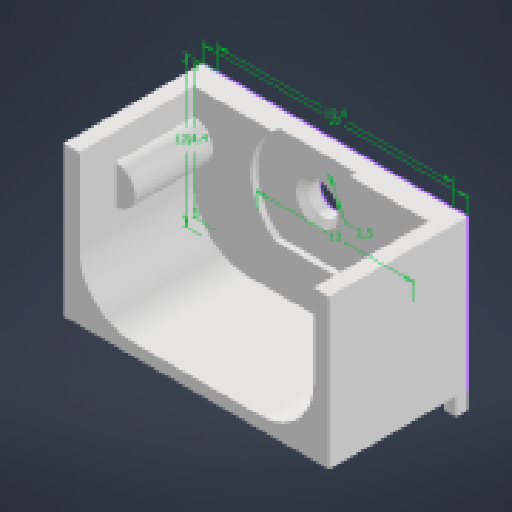
# Autodesk Inventor part: MotorHolder
Saved by Autodesk Inventor 2024 (Build 280153000, 153)
## iProperties
Created: 2023-10-23
Part Number: MotorHolder
Material: Generic
Document SubType Name: Modeling
Designer: 21guslof
Density: 1 g/cm^3
Appearance: Default
Author: 21guslof
Autodesk Inventor part; units mm, degrees
ref_plane "YZ Plane" through (0, 0, 0) normal (1, 0, 0) x (0, 1, 0)
ref_plane "XZ Plane" through (0, 0, 0) normal (0, 1, 0) x (-1, 0, 0)
ref_plane "XY Plane" through (0, 0, 0) normal (0, 0, 1) x (1, 0, 0)
sketch "Sketch1" plane through (0, 0, 0) normal (0, 0, 1) x (1, 0, 0)
  line L0 (9.7, 0) -> (-9.7, 0)
  line L1 (-9.7, 0) -> (-9.7, 11.4)
  line L2 (-9.7, 11.4) -> (9.7, 11.4)
  line L3 (9.7, 11.4) -> (9.7, 0)
  line L4 (-9.7, 6) -> (-9.7, 0)
  line L5 (-9.7, 0) -> (9.7, 0)
  line L6 (9.7, 0) -> (9.7, 6)
  arc A0 (-9.7, 6) -> (-9.7, 9.2) centre (-9.7, 7.6) ccw
  arc A1 (9.7, 9.2) -> (9.7, 6) centre (9.7, 7.6) ccw
  line L7 (6.5, 0) -> (-6.5, 0)
  line L8 (-6.5, 0) -> (-6.5, 3)
  line L9 (-6.5, 3) -> (6.5, 3)
  line L10 (6.5, 3) -> (6.5, 0)
  line L11 (2.9833, 3.65) -> (-2.9833, 3.65)
  line L12 (-3.1721, 11.4) -> (3.1721, 11.4)
  arc A2 (-3.1721, 11.4) -> (-2.9833, 3.65) centre (0, 7.6) ccw
  arc A3 (2.9833, 3.65) -> (3.1721, 11.4) centre (0, 7.6) ccw
  circle A4 centre (0, 7.6) radius 1.25
  line L13 (11, -1) -> (-11, -1)
  line L14 (-11, -1) -> (-11, 11.4)
  line L15 (-11, 11.4) -> (11, 11.4)
  line L16 (11, 11.4) -> (11, -1)
  point P0 (0, 0)
  dimension "d0" = 19.4
  dimension "d1" = 11.4
  dimension "d3" = 13
  dimension "d5" = 2.5
  dimension "d6" = 22
  dimension "d7" = 12.4
  constraints: 34 end point, 8 point on circle, 7 parallel, 6 point on line, 5 centre point, 3 horizontal, 3 perpendicular, 1 coincident
  measures "d0" distance of L1.end L2.end
  measures "d1" distance of L0.end L1.end
  measures "d3" distance of L8.end L9.end
  measures "d5" diameter of A4
  measures "d6" distance of L14.end L15.end
  measures "d7" distance of L13.end L14.end
extrude "Extrusion1" add sketch "Sketch1" along normal blind 10 contours L3 L15 L16 L13 L14 L1 L0
extrude "Extrusion3" add sketch "Sketch1" along normal blind 8.5 contours A1 L3 | L1 A0
extrude "Extrusion4" add sketch "Sketch1" along normal blind 1.5 contours L0 L10 L9 L8 L1 A0 L2 A2 L11 A3 L3 A1 | L0 L8 L9 L10 | A3 L11 A2 L2
chamfer "Chamfer1" distance 0.5 angle 45 1 edges at (-1.25, 7.6, 1.5)
fillet "Fillet1" radius 4.5 2 edges at (-9.7, 0, 5.75) (9.7, 0, 5.75)
extrude "Extrusion6" add sketch "Sketch1" along normal blind 2 contours L0 L10 L9 L8 L1 A0 L2 A2 L11 A3 L3 A1 | L0 L8 L9 L10
move faces "Move1" translate (0, 0, 1.5) faces at (-1.7333, -0.6667, 10)
sketch "Sketch2" plane through (-11, -1, 0) normal (0, -1, 0) x (1, 0, 0)
  line L0 (22, 0) -> (22, 11.5) projected
  line L1 (0, 0) -> (22, 0)
  line L2 (22, 0) -> (22, 1)
  line L3 (22, 1) -> (0, 1)
  line L4 (0, 1) -> (0, 0)
  line L5 (5, 0) -> (4.6249, 0)
  line L6 (4.6249, 1) -> (5, 1)
  line L7 (0, 0) -> (22, 0) projected
  line L8 (17, 0) -> (17, 1)
  line L9 (5, 0) -> (5, 1)
  line L10 (1, 0) -> (1, 1)
  line L11 (21, 0) -> (21, 1)
  point P0 (11, 0)
  point P1 (0, 0.5)
  point P2 (4.9955, 0.5057)
  point P3 (5, 0.5)
  point P4 (21, 0.5)
  point P5 (1, 0)
  dimension "d28" = 1
  dimension "d30" = 5
  dimension "d31" = 5
  dimension "d32" = 1
  dimension "d33" = 1
  constraints: 20 end point, 7 point on line, 5 perpendicular, 3 midpoint, 3 parallel, 2 horizontal, 5 other
  measures "d28" distance of L2.end L1.end
  measures "d30" distance between parallel lines of L0 L8
  measures "d31" distance from line of point (5, 0.5) L4
  measures "d32" distance from line of point (21, 0.5) L0
  measures "d33" distance between parallel lines of L4 L10
extrude "Extrusion7" add sketch "Sketch2" along normal blind 1.5 contours L1 L11 L3 L0 | L1 L9 L3 L8 | L1 L4 L3 L10
body "Solid1"
